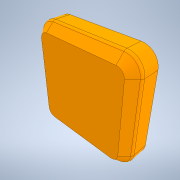
# Autodesk Inventor part: Колпачок датчика
Saved by Autodesk Inventor 2021.1 (Build 251245010, 245A)
## iProperties
Created: 2026-06-02
Part Number: Колпачок датчика
Material: Типовые
Document SubType Name: Modeling
Designer: Андрей Тарасов
Density: 1 g/cm^3
Appearance: По умолчанию
Author: Андрей Тарасов
Autodesk Inventor part; units mm, degrees
ref_plane "YZ Plane" through (0, 0, 0) normal (1, 0, 0) x (0, 1, 0)
ref_plane "XZ Plane" through (0, 0, 0) normal (0, 1, 0) x (-1, 0, 0)
ref_plane "XY Plane" through (0, 0, 0) normal (0, 0, 1) x (1, 0, 0)
sketch "Эскиз1" plane through (0, 0, 0) normal (0, 0, 1) x (1, 0, 0)
  line L0 (8.55, -11.55) -> (-8.55, -11.55)
  line L1 (-11.55, -8.55) -> (-11.55, 8.55)
  line L2 (-8.55, 11.55) -> (8.55, 11.55)
  line L3 (11.55, 8.55) -> (11.55, -8.55)
  line L4 (11.55, -11.55) -> (-11.55, 11.55) construction
  line L5 (-11.55, -11.55) -> (11.55, 11.55) construction
  arc A0 (-8.55, 11.55) -> (-11.55, 8.55) centre (-8.55, 8.55) ccw
  arc A1 (11.55, 8.55) -> (8.55, 11.55) centre (8.55, 8.55) ccw
  arc A2 (-11.55, -8.55) -> (-8.55, -11.55) centre (-8.55, -8.55) ccw
  arc A3 (8.55, -11.55) -> (11.55, -8.55) centre (8.55, -8.55) ccw
  line L6 (8.55, 12.35) -> (-8.55, 12.35)
  arc A4 (-8.55, 12.35) -> (-12.35, 8.55) centre (-8.55, 8.55) ccw
  line L7 (-12.35, 8.55) -> (-12.35, -8.55)
  arc A5 (-12.35, -8.55) -> (-8.55, -12.35) centre (-8.55, -8.55) ccw
  line L8 (-8.55, -12.35) -> (8.55, -12.35)
  arc A6 (8.55, -12.35) -> (12.35, -8.55) centre (8.55, -8.55) ccw
  line L9 (12.35, -8.55) -> (12.35, 8.55)
  arc A7 (12.35, 8.55) -> (8.55, 12.35) centre (8.55, 8.55) ccw
  point P0 (0, 0)
  dimension "d0" = 23.1
  dimension "d1" = 3
  dimension "d2" = 0.8
  constraints: 20 end point, 16 point on circle, 8 centre point, 8 point on line, 8 tangent, 4 parallel, 3 equal radius, 3 perpendicular, 2 midpoint, 1 horizontal, 7 other
  measures "d0" distance of L5.start L4.end
  measures "d1" radius of A0
  measures "d2" distance between parallel lines of L2 L6
extrude "Выдавливание1" add sketch "Эскиз1" along normal blind 6 contours L0 A2 L1 A0 L2 A1 L3 A3 | A7 L9 A6 L8 A5 L7 A4 L6
chamfer "Фаска1" distance 2 angle 45 8 edges at (0, 12.35, 6) (-11.237, 11.237, 6) (-12.35, 0, 6) (-11.237, -11.237, 6) (0, -12.35, 6) (11.237, -11.237, 6) (12.35, 0, 6) (11.237, 11.237, 6)
shell "Оболочка1" thickness 0.8 removed faces 1 at (2.85, -4.1167, 0)
sketch "Эскиз3" plane through (0, 0, 0) normal (0, 0, -1) x (-1, 0, 0)
  line L0 (14.85, -2.5) -> (9.85, -2.5)
  line L1 (9.85, -2.5) -> (9.85, 2.5)
  line L2 (9.85, 2.5) -> (14.85, 2.5)
  line L3 (14.85, 2.5) -> (14.85, -2.5)
  line L4 (12.35, 8.55) -> (12.35, -8.55) projected
  line L5 (14.85, -2.5) -> (9.85, 2.5) construction
  line L6 (9.85, -2.5) -> (14.85, 2.5) construction
  point P0 (0, 0)
  point P1 (12.35, 0)
  dimension "d11" = 5
  dimension "d12" = 5
  constraints: 12 end point, 3 midpoint, 2 parallel, 1 horizontal, 1 perpendicular
  measures "d11" distance of L1.end L2.end
  measures "d12" distance of L0.end L1.end
extrude "Выдавливание3" cut sketch "Эскиз3" against normal blind 5
fillet "Сопряжение1" radius 1 20 edges at (-11.237, -11.237, 4) (0, -12.35, 4) (11.237, -11.237, 4) (12.35, 0, 4) (11.237, 11.237, 4) (0, 12.35, 4) (-11.237, 11.237, 4) (-12.35, 5.525, 4) (-12.35, -5.525, 4) (-10.6713, 10.6713, 3.6686) (0, 11.55, 3.6686) (10.6713, 10.6713, 3.6686) (11.55, 0, 3.6686) (10.6713, -10.6713, 3.6686) (0, -11.55, 3.6686) (-10.6713, -10.6713, 3.6686) (-11.55, -5.525, 3.6686) (-11.55, 5.525, 3.6686) (-10.7843, 2.5, 5) (-10.7843, -2.5, 5)
fillet "Сопряжение2" radius 0.4 16 edges at (-11.4739, 2.5, 3.6371) (-10.5115, 2.2071, 4.7071) (-10.2186, 0, 5) (-10.5115, -2.2071, 4.7071) (-11.4739, -2.5, 3.6371) (-11.55, -2.5, 1.6272) (-11.55, 2.5, 1.6272) (-12.3273, 2.5, 3.7977) (-12.1711, 2.4877, 4.1565) (-11.546, 2.0946, 4.804) (-11.35, 0, 5) (-11.546, -2.0946, 4.804) (-12.1711, -2.4877, 4.1565) (-12.3273, -2.5, 3.7977) (-12.35, -2.5, 1.7929) (-12.35, 2.5, 1.7929)
